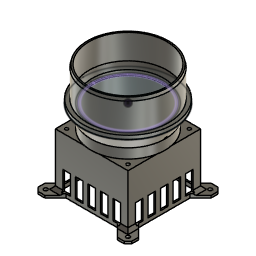
fanhousing v2 (Autodesk Fusion 360 design; units mm, degrees)
Autodesk Fusion 360 part; units mm, degrees
sketch "Sketch1" plane through (0, 0, 0) normal (0, 0, 1) x (1, 0, 0)
  line L0 (46.5, -46.5) -> (-46.5, -46.5)
  line L1 (-46.5, -46.5) -> (-46.5, 46.5)
  line L2 (-46.5, 46.5) -> (46.5, 46.5)
  line L3 (46.5, 46.5) -> (46.5, -46.5)
  line L4 (46.5, -46.5) -> (-46.5, 46.5)
  line L5 (48.5, -48.5) -> (-48.5, -48.5)
  line L6 (-48.5, -48.5) -> (-48.5, 48.5)
  line L7 (-48.5, 48.5) -> (48.5, 48.5)
  line L8 (48.5, 48.5) -> (48.5, -48.5)
  circle A0 centre (0, 0) radius 45
  circle A1 centre (0, 0) radius 47
  circle A2 centre (41, -41) radius 2.15
  circle A3 centre (-41, -41) radius 2.15
  circle A4 centre (-41, 41) radius 2.15
  circle A5 centre (41, 41) radius 2.15
  line L9 (0, -48.5) -> (0, 48.5)
  line L10 (48.5, 0) -> (-48.5, 0)
  line L11 (41, -41) -> (0, -41) construction
  line L12 (0, -41) -> (-41, -41) construction
  line L13 (41, -41) -> (41, 0) construction
  line L14 (41, 0) -> (41, 41) construction
  line L15 (41, 41) -> (0, 41) construction
  line L16 (0, 41) -> (-41, 41) construction
  line L17 (-41, 41) -> (-41, 0) construction
  line L18 (-41, -41) -> (-41, 0) construction
  dimension "d1" = 93
  dimension "d2" = -2
  dimension "d3" = 90
  dimension "d4" = 94
  dimension "d5" = 4.3
  dimension "d6" = 82
  dimension "d7" = 82
  dimension "d8" = 82
  constraint horizontal L0
  constraint vertical L1
  constraint horizontal L2
  constraint vertical L3
  constraint equal L0 L3
  constraint midpoint A0.centre L4
  constraint coincident A0.centre A1.centre
  constraint concentric A0 A1
  constraint coincident L4 A2.centre
  constraint coincident L4 A4.centre
  constraint equal A2 A3
  constraint equal A3 A4
  constraint equal A4 A5
  constraint midpoint L5 L9.start
  constraint midpoint L7 L9.end
  constraint midpoint L8 L10.start
  constraint midpoint L6 L10.end
  constraint coincident A2.centre L11.start
  constraint coincident L9 L11.end
  constraint perpendicular L9 L11
  constraint coincident A3.centre L12.end
  constraint parallel L11 L12
  constraint equal L11 L12
  constraint coincident L10 L13.end
  constraint perpendicular L10 L13
  constraint coincident A5.centre L14.end
  constraint coincident L9 L15.end
  constraint perpendicular L9 L15
  constraint coincident A4.centre L16.end
  constraint parallel L15 L16
  constraint coincident L10 L17.end
  constraint perpendicular L10 L17
  constraint perpendicular L10 L18
  measures "d1" distance of L0.start L0.end
  measures "d3" diameter of A0
  measures "d4" diameter of A1
  measures "d5" diameter of A2
  measures "d6" distance of A2.centre A3.centre
  measures "d7" distance of A4.centre A5.centre
  measures "d8" vertical distance of A3.centre A4.centre
extrude "Extrude1" add sketch "Sketch1" along normal blind 103 contours L0 A1 L9 | L0 L4 A0 A1 L9 | L3 L4 A0 A1 L10 | L3 A1 L10 | L0 A1 L9 | L0 L1 A0 A1 L9 L10 | L2 L3 A0 A1 L9 L10 | L3 A1 L10 | L1 A1 L10 | L1 L4 A0 A1 L10 | L2 A1 L9 | L2 L4 A0 A1 L9 | L1 A1 L10 | L2 A1 L9 makes body 1
extrude "Extrude2" add sketch "Sketch1" along normal blind 73 contours L0 L3 L5 L8 A1 L9 L10 | L3 L4 A1 A2 | L0 L4 A1 A2 | L0 L1 L5 L6 A1 L9 L10 | L2 L3 L7 L8 A1 L9 L10 | L0 L1 A1 | L2 L3 A1 | L1 L2 L6 L7 A1 L9 L10 | L1 L4 A1 A4 | L2 L4 A1 A4 bodies 1
extrude "Extrude3" cut sketch "Sketch1" along normal blind 70 contours L3 L4 A1 A2 | L0 L4 A1 A2 | L0 L4 A0 A1 L9 | L3 L4 A0 A1 L10 | L0 L1 A0 A1 L9 L10 | L2 L3 A0 A1 L9 L10 | L0 L1 A1 | L2 L3 A1 | L1 L4 A0 A1 L10 | L2 L4 A0 A1 L9 | L1 L4 A1 A4 | L2 L4 A1 A4 bodies 1
sketch "Sketch2" plane through (48.5, 0, 0) normal (1, 0, 0) x (0, 1, 0)
  line L0 (-48.5, 0) -> (48.5, 0)
  line L1 (48.5, 0) -> (48.5, 73)
  line L2 (48.5, 73) -> (-48.5, 73)
  line L3 (-48.5, 73) -> (-48.5, 0)
  line L4 (-48.5, 5) -> (48.5, 5) construction
  line L5 (-38.5, 73) -> (-38.5, 0) construction
  line L6 (38.5, 73) -> (38.5, 0) construction
  line L7 (48.5, 0) -> (-48.5, 0)
  line L8 (-48.5, 31) -> (48.5, 31) construction
  line L9 (-38.5, 31) -> (-28.5, 31)
  line L10 (-28.5, 31) -> (-28.5, 5)
  line L11 (-28.5, 5) -> (-38.5, 5)
  line L12 (-38.5, 5) -> (-38.5, 31)
  line L13 (38.5, 31) -> (28.5, 31)
  line L14 (28.5, 31) -> (28.5, 5)
  line L15 (28.5, 5) -> (38.5, 5)
  line L16 (38.5, 5) -> (38.5, 31)
  line L17 (-5, 5) -> (5, 5)
  line L18 (5, 5) -> (5, 31)
  line L19 (5, 31) -> (-5, 31)
  line L20 (-5, 31) -> (-5, 5)
  line L21 (-28.5, 5) -> (-5, 5) construction
  line L22 (5, 5) -> (28.5, 5) construction
  line L23 (-21.75, 31) -> (-11.75, 31)
  line L24 (-11.75, 31) -> (-11.75, 5)
  line L25 (-11.75, 5) -> (-21.75, 5)
  line L26 (-21.75, 5) -> (-21.75, 31)
  line L27 (11.75, 5) -> (21.75, 5)
  line L28 (21.75, 5) -> (21.75, 31)
  line L29 (21.75, 31) -> (11.75, 31)
  line L30 (11.75, 31) -> (11.75, 5)
  point P0 (0, 5)
  dimension "d15" = 10
  dimension "d16" = 10
  dimension "d17" = 5
  dimension "d18" = 42
  dimension "d19" = 10
  dimension "d20" = 10
  dimension "d21" = 10
  dimension "d22" = 10
  dimension "d23" = 10
  constraint coincident L3 L4.start
  constraint coincident L1 L4.end
  constraint perpendicular L1 L4
  constraint coincident L2 L5.start
  constraint coincident L0 L5.end
  constraint perpendicular L0 L5
  constraint coincident L2 L6.start
  constraint coincident L0 L6.end
  constraint perpendicular L0 L6
  constraint coincident L3 L8.start
  constraint coincident L1 L8.end
  constraint perpendicular L1 L8
  constraint horizontal L9
  constraint vertical L10
  constraint horizontal L11
  constraint vertical L12
  constraint coincident L4 L10.end
  constraint coincident L5 L9.start
  constraint coincident L8 L9.start
  constraint horizontal L13
  constraint vertical L14
  constraint horizontal L15
  constraint vertical L16
  constraint coincident L8 L13.start
  constraint coincident L6 L13.start
  constraint midpoint L4 P0
  constraint horizontal L17
  constraint vertical L18
  constraint horizontal L19
  constraint vertical L20
  constraint coincident L4 L17.start
  constraint midpoint P0 L17
  constraint perpendicular L14 L22
  constraint horizontal L23
  constraint vertical L24
  constraint horizontal L25
  constraint vertical L26
  constraint coincident L8 L23.start
  constraint horizontal L27
  constraint vertical L28
  constraint horizontal L29
  constraint vertical L30
  constraint coincident L8 L28.end
  constraint coincident L22 L27.start
  constraint midpoint L22 L27
  constraint midpoint L21 L25
  measures "d15" distance of L3 L5
  measures "d16" distance of L1 L6
  measures "d17" distance of L4 L7
  measures "d18" distance of L2 L8
  measures "d19" distance of L9.start L9.end
  measures "d20" distance of L13.start L13.end
  measures "d21" distance of L17.start L17.end
  measures "d22" distance of L23.start L23.end
  measures "d23" distance of L28.end L29.end
extrude "Extrude4" cut sketch "Sketch2" against normal blind 2 contours L9 L10 L11 L12 | L13 L14 L15 L16 | L17 L18 L19 L20 | L23 L24 L25 L26 | L27 L28 L29 L30 bodies 1
pattern_circular "C-Pattern1" count 4 over 360 about axis through (0, 0, 1.75) along (0, 0, 1) of "Extrude4"
sketch "Sketch3" plane through (0, 0, 0) normal (0, 0, 1) x (1, 0, 0)
  circle A0 centre (41, -41) radius 2.15
  circle A1 centre (41, 41) radius 2.15
  circle A2 centre (-41, 41) radius 2.15
  circle A3 centre (0, 0) radius 45
  circle A4 centre (-41, -41) radius 2.15
  line L0 (48.5, 48.5) -> (48.5, -48.5)
  line L1 (48.5, -48.5) -> (-48.5, -48.5)
  line L2 (-48.5, -48.5) -> (-48.5, 48.5)
  line L3 (-48.5, 48.5) -> (48.5, 48.5)
  line L4 (34.3579, -48.5) -> (48.5, -62.6421)
  line L5 (34.3579, -48.5) -> (54.3579, -48.5) construction
  line L6 (48.5, -48.5) -> (69.3401, -69.3401) construction
  line L7 (48.5, -48.5) -> (77.9723, -48.5) construction
  line L8 (48.5, -62.6421) -> (62.6421, -62.6421)
  circle A5 centre (55, -55) radius 2.5
  line L9 (48.5, -34.3579) -> (62.6421, -48.5)
  line L10 (62.6421, -48.5) -> (62.6421, -62.6421)
  dimension "d28" = 20
  dimension "d29" = 45
  dimension "d30" = 45
  dimension "d31" = 10
  dimension "d32" = 5
  constraint horizontal L5
  constraint coincident L1 L4.start
  constraint horizontal L7
  constraint coincident L0.end L1.start
  constraint coincident L6 L8.end
  constraint horizontal L8
  constraint coincident L6 A5.centre
  constraint symmetric L4.start L6 L9.start
  constraint symmetric L4.end L6 L9.end
  constraint symmetric L6 L8.end L10.end
  measures "d28" distance of L4.start L4.end
  measures "d29" angle of L4 L5
  measures "d30" angle of L6 L7
  measures "d31" distance of L4 L6
  measures "d32" diameter of A5
extrude "Extrude5" add sketch "Sketch3" along normal blind 3 contours L0 L1 L4 L8 L9 L10 bodies 1
pattern_circular "C-Pattern2" count 4 over 360 about axis through (0, 0, 1.75) along (0, 0, 1) of "Extrude5"
chamfer "Chamfer1" distance 4 angle 45 8 edges at (41.4289, -48.5, 3) (48.5, -41.4289, 3) (48.5, 41.4289, 3) (41.4289, 48.5, 3) (-41.4289, 48.5, 3) (-48.5, 41.4289, 3) (-48.5, -41.4289, 3) (-41.4289, -48.5, 3) on bodies 1
chamfer "Chamfer2" distance 5 angle 45 4 edges at (62.6421, -62.6421, 1.5) (-62.6421, -62.6421, 1.5) (-62.6421, 62.6421, 1.5) (62.6421, 62.6421, 1.5) on bodies 1
sketch "Sketch1 (2)" plane through (0, 0, 103) normal (0, 0, 1) x (-1, 0, 0) in component "adapter"
  circle A0 centre (0, 0) radius 45
  circle A1 centre (0, 0) radius 47
  circle A2 centre (0, 0) radius 47.5
  circle A3 centre (0, 0) radius 49.5
  circle A4 centre (0, 0) radius 60
  dimension "d39" = 0.5
  dimension "d40" = 2.5
  dimension "d41" = 120
  constraint concentric A0 A4
  measures "d41" diameter of A4
extrude "Extrude1'" add sketch "Sketch1 (2)" against normal blind 30 separate body contours A3 makes body 2 in component "adapter"
extrude "Extrude2'" add sketch "Sketch1 (2)" along normal blind 5 contours A3 | A4 bodies 2 in component "adapter"
chamfer "Chamfer1'" distance 10.5 distance2 17 1 edges at (46.1502, 17.9, 103) measured on face at (-56.0923, 5.44, 103) on bodies 2 in component "adapter"
sketch "Sketch2 (2)" plane through (0, 0, 108) normal (0, 0, 1) x (-1, 0, 0) in component "adapter"
  circle A0 centre (0, 0) radius 47.5
  circle A1 centre (0, 0) radius 60
  circle A2 centre (0, 0) radius 55
  circle A3 centre (0, 0) radius 52
  dimension "d48" = 110
  dimension "d49" = -3
  constraint concentric A0 A2
  measures "d48" diameter of A2
extrude "Extrude3'" add sketch "Sketch2 (2)" along normal blind 40 contours A2 bodies 2 in component "adapter"
chamfer "Chamfer2'" distance 1 distance2 4 1 edges at (51.278, 19.8888, 148) measured on face at (-53.7952, 2.7324, 148) on bodies 2 in component "adapter"
chamfer "Chamfer3" distance 4.5 distance2 7 1 edges at (48.481, 18.804, 108) measured on face at (-50.1296, 4.9432, 108) on bodies 2 in component "adapter"
sketch "Sketch3 (2)" plane through (0, 0, 0) normal (1, 0, 0) x (0, 1, 0) in component "adapter"
  line L0 (-54, 148) -> (54, 148)
  line L1 (60, 108) -> (55, 108)
  line L2 (-55, 108) -> (-60, 108)
  line L3 (-49.5, 73) -> (49.5, 73)
  line L4 (-54, 148) -> (-55, 144)
  line L5 (54, 148) -> (55, 144)
  line L6 (55, 108) -> (55, 144)
  line L7 (-55, 108) -> (-55, 144)
  line L8 (49.5, 86) -> (60, 103)
  line L9 (-49.5, 86) -> (-60, 103)
  line L10 (-49.5, 86) -> (-49.5, 73)
  line L11 (49.5, 86) -> (49.5, 73)
  line L12 (60, 103) -> (60, 108)
  line L13 (-60, 103) -> (-60, 108)
  line L14 (0, 103) -> (0, 73) construction
  circle A0 centre (0, 88) radius 2
  point P0 (0, 103)
  dimension "d56" = 4
  constraint coincident P0 L14.start
  constraint midpoint L3 L14.end
  constraint perpendicular L3 L14
  constraint midpoint L14 A0.centre
  measures "d56" diameter of A0
extrude "Extrude6" cut sketch "Sketch3 (2)" along normal through all and the other way through all contours A0 bodies 1
extrude "Extrude4'" cut sketch "Sketch3 (2)" along normal through all and the other way through all contours A0 bodies 2 in component "adapter"
component "adapter" placed x (1, 0, 0) y (0, 1, 0) z (0, 0, 1) at (0, 0, 0)
equation "d9 = 70 mm + 3 mm + 30 mm"
